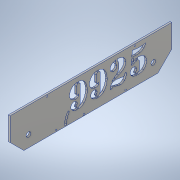
# Autodesk Inventor part: DriveTrain3.0
Saved by Autodesk Inventor 2021 (Build 250183000, 183)
## iProperties
Created: 2017-07-22
Part Number: DriveTrain3.0
Material: Aluminum 6061
Document SubType Name: Modeling
Designer: User
Density: 2.7 g/cm^3
Appearance: Aluminum - Flat
Mass: 590.045 g
Surface Area: 982.684 cm^2
Volume: 218.535 cm^3
Author: User
Autodesk Inventor part; units mm, degrees
ref_plane "YZ Plane" through (0, 0, 0) normal (1, 0, 0) x (0, 1, 0)
ref_plane "XZ Plane" through (0, 0, 0) normal (0, 1, 0) x (-1, 0, 0)
ref_plane "XY Plane" through (0, 0, 0) normal (0, 0, 1) x (1, 0, 0)
sketch "Sketch1" plane through (0, 0, 0) normal (1, 0, 0) x (0, 1, 0)
  line L0 (0, 0) -> (101.6, 0)
  line L1 (101.6, 0) -> (101.6, -444.5)
  line L2 (101.6, -444.5) -> (0, -444.5)
  line L3 (0, -444.5) -> (0, 0)
  circle A0 centre (31.75, -50.8) radius 6.3627
  circle A1 centre (31.75, -393.7) radius 6.3627
  circle A2 centre (86.2838, -165.5318) radius 1.5875
  circle A3 centre (70.2818, -165.5318) radius 1.5875
  circle A4 centre (15.3162, -278.9682) radius 1.5875
  circle A5 centre (31.3182, -278.9682) radius 1.5875
  dimension "d0" = 101.6
  dimension "d1" = 444.5
  dimension "d2" = 12.7254
  dimension "d3" = 31.75
  dimension "d4" = 50.8
  dimension "d5" = 50.8
  dimension "d22" = 165.5318
  dimension "d23" = 3.175
  dimension "d24" = 15.3162
  dimension "d25" = 3.175
  dimension "d26" = 16.002
  dimension "d27" = 165.5318
  dimension "d28" = 3.175
  dimension "d29" = 15.3162
  dimension "d30" = 165.5318
  dimension "d31" = 3.175
  dimension "d32" = 16.002
  dimension "d33" = 165.5318
  constraints: 8 end point, 6 centre point, 2 parallel, 1 horizontal, 1 perpendicular
  measures "d0" distance of L1.end L2.end
  measures "d1" distance of L0.end L1.end
  measures "d2" diameter of A0
  measures "d3" distance from line of L3 A0.centre
  measures "d4" distance from line of L0 A0.centre
  measures "d5" distance from line of L2 A1.centre
  measures "d22" distance from line of L0 A2.centre
  measures "d23" diameter of A2
  measures "d24" distance from line of L1 A2.centre
  measures "d25" diameter of A3
  measures "d26" distance of A2.centre A3.centre
  measures "d27" distance from line of L0 A3.centre
  measures "d28" diameter of A4
  measures "d29" distance from line of L3 A4.centre
  measures "d30" distance from line of L2 A4.centre
  measures "d31" diameter of A5
  measures "d32" distance of A5.centre A4.centre
  measures "d33" distance from line of L2 A5.centre
extrude "Extrusion1" add sketch "Sketch1" along normal blind 4.7625 contours L0 L1 L2 L3 | A2 | A3 | A4 | A5
chamfer "Chamfer1" distance 38.1 angle 45 1 edges at (2.3813, 0, 0)
chamfer "Chamfer2" distance 38.1 angle 45 1 edges at (2.3813, 0, -444.5)
sketch "Sketch8" plane through (4.7625, 0, 0) normal (1, 0, 0) x (0, 0, -1)
  line L0 (444.5, 38.1) -> (406.4, 0) projected
  line L1 (444.5, 38.1) -> (444.5, 101.6) projected
  line L2 (444.5, 101.6) -> (0, 101.6) projected
  line L3 (0, 101.6) -> (0, 38.1) projected
  line L4 (38.1, 0) -> (0, 38.1) projected
  line L5 (38.1, 0) -> (406.4, 0) projected
  circle A0 centre (393.7, 31.75) radius 6.3627 projected
  circle A1 centre (50.8, 31.75) radius 6.3627 projected
  point P0 (0, 0)
  point P1 (101.6, 97.155)
  point P2 (342.9, 97.155)
  point P3 (127, 4.445)
  point P4 (317.5, 4.445)
  dimension "d110" = 4.445
  dimension "d111" = 4.445
  dimension "d112" = 101.6
  dimension "d113" = 101.6
  dimension "d114" = 4.445
  dimension "d115" = 4.445
  dimension "d123" = 127
  dimension "d124" = 127
  measures "d110" distance from line of L2 point (342.9, 97.155)
  measures "d111" distance from line of L2 point (101.6, 97.155)
  measures "d112" distance from line of L3 point (101.6, 97.155)
  measures "d113" distance from line of L1 point (342.9, 97.155)
  measures "d114" distance from line of L5 point (317.5, 4.445)
  measures "d115" distance from line of L5 point (127, 4.445)
  measures "d123" distance from line of L1 point (317.5, 4.445)
  measures "d124" distance from line of L3 point (127, 4.445)
hole "Hole3" at (4.7625, 97.155, -101.6) at (4.7625, 97.155, -342.9) at (4.7625, 4.445, -127) at (4.7625, 4.445, -317.5) direction (-1, 0, 0) diameter 3.81 depth 25.4 tip angle 118
sketch "Sketch9" plane through (4.7625, 0, 0) normal (1, 0, 0) x (0, 0, -1)
  line L0 (444.5, 38.1) -> (444.5, 101.6) projected
  line L1 (38.1, 0) -> (406.4, 0) projected
  arc A0 (159.964, 30.48) -> (152.4159, 5.08) centre (203.2, 3.81) ccw construction
  arc A1 (157.8022, 31.8135) -> (149.8767, 5.1435) centre (203.2, 3.81) ccw
  arc A2 (162.1258, 29.1465) -> (154.9551, 5.0165) centre (203.2, 3.81) ccw
  arc A3 (162.1258, 29.1465) -> (157.8022, 31.8135) centre (159.964, 30.48) ccw
  arc A4 (149.8767, 5.1435) -> (154.9551, 5.0165) centre (152.4159, 5.08) ccw
  line L2 (0, 101.6) -> (0, 38.1) projected
  point P0 (0, 0)
  dimension "d126" = 3.81
  dimension "d134" = 50.8
  dimension "d135" = 5.08
  dimension "d238" = 203.2
  dimension "d239" = 5.08
  dimension "d240" = 25.4
  constraints: 10 point on circle, 5 centre point, 4 tangent, 1 coincident
  measures "d126" distance from line of point (203.2, 3.81) L1
  measures "d134" radius of A0
  measures "d135" diameter of A4
  measures "d238" distance from line of L2 point (203.2, 3.81)
  measures "d239" distance from line of A0.end L1
  measures "d240" vertical distance of A0.end A0.start
hole "Hole4" at (4.7625, 3.81, -203.2) direction (-1, 0, 0) diameter 5.08 end through all
extrude "Extrusion6" cut sketch "Sketch9" against normal through all
sketch "Sketch10" plane through (4.7625, 0, 0) normal (1, 0, 0) x (0, 0, -1)
  line L0 (161.1896, 89.2474) -> (414.9055, 89.2474) construction
  line L1 (414.9055, 89.2474) -> (414.9055, 0) construction
  line L2 (414.9055, 0) -> (161.1896, 0) construction
  line L3 (161.1896, 0) -> (161.1896, 89.2474) construction
  line L4 (188.4748, 24.204) -> (188.4748, 28.8893)
  spline S0 degree 2 poles (188.4748, 28.8893) (189.963, 29.3303) (191.5064, 30.3776) (192.0577, 31.3698) knots 0 0 0 1 2 2 2
  spline S1 degree 2 poles (192.0577, 31.3698) (193.2152, 33.299) (193.2152, 35.6141) knots 0 0 0 1 1 1
  line L5 (193.2152, 35.6141) -> (193.2152, 78.5538)
  spline S2 degree 2 poles (193.2152, 78.5538) (193.2152, 80.7036) (192.9396, 82.5226) (192.4435, 83.184) knots 0 0 0 1 2 2 2
  spline S3 degree 2 poles (192.4435, 83.184) (191.6718, 84.1211) (189.5772, 84.7274) knots 0 0 0 1 1 1
  line L6 (189.5772, 84.7274) -> (189.5772, 89.2474)
  spline S4 degree 2 poles (189.5772, 89.2474) (194.042, 88.8064) (201.8693, 84.4518) (204.901, 80.7587) knots 0 0 0 1 2 2 2
  spline S5 degree 2 poles (204.901, 80.7587) (208.3736, 76.6797) (212.1219, 63.8364) (212.1219, 56.3398) knots 0 0 0 1 2 2 2
  spline S6 degree 2 poles (212.1219, 56.3398) (212.1219, 40.3546) (202.9717, 31.0391) knots 0 0 0 1 1 1
  spline S7 degree 2 poles (202.9717, 31.0391) (199.7195, 27.7869) (192.1679, 24.204) (188.4748, 24.204) knots 0 0 0 1 2 2 2
  line L7 (189.5772, 59.3715) -> (189.5772, 54.0247)
  spline S8 degree 2 poles (189.5772, 54.0247) (184.506, 51.2687) (179.7656, 51.2687) knots 0 0 0 1 1 1
  spline S9 degree 2 poles (179.7656, 51.2687) (176.8441, 51.2687) (171.0564, 53.5286) (168.8515, 55.4579) knots 0 0 0 1 2 2 2
  spline S10 degree 2 poles (168.8515, 55.4579) (166.4261, 57.6628) (163.7252, 64.0569) (163.7252, 67.6949) knots 0 0 0 1 2 2 2
  spline S11 degree 2 poles (163.7252, 67.6949) (163.7252, 72.8763) (168.5208, 82.5777) (172.4895, 85.3338) knots 0 0 0 1 2 2 2
  spline S12 degree 2 poles (172.4895, 85.3338) (178.2221, 89.2474) (186.0494, 89.2474) knots 0 0 0 1 1 1
  line L8 (186.0494, 89.2474) -> (186.0494, 84.7274)
  spline S13 degree 2 poles (186.0494, 84.7274) (184.2304, 84.2313) (182.6319, 82.1918) (182.6319, 80.2075) knots 0 0 0 1 2 2 2
  line L9 (182.6319, 80.2075) -> (182.6319, 62.5134)
  spline S14 degree 2 poles (182.6319, 62.5134) (182.6319, 60.4188) (184.3958, 58.0486) (185.884, 58.1037) knots 0 0 0 1 2 2 2
  spline S15 degree 2 poles (185.884, 58.1037) (187.3172, 58.1588) (189.5772, 59.3715) knots 0 0 0 1 1 1
  line L10 (185.0021, 28.8893) -> (185.0021, 24.204)
  spline S16 degree 2 poles (185.0021, 24.204) (180.3719, 24.204) (175.6314, 26.4088) knots 0 0 0 1 1 1
  spline S17 degree 2 poles (175.6314, 26.4088) (171.6627, 28.3381) (167.1427, 34.4015) (167.1427, 37.9292) knots 0 0 0 1 2 2 2
  spline S18 degree 2 poles (167.1427, 37.9292) (167.1427, 41.7878) (172.3241, 47.0243) (176.2378, 47.0243) knots 0 0 0 1 2 2 2
  spline S19 degree 2 poles (176.2378, 47.0243) (179.7104, 47.0243) (184.5611, 42.5043) (184.5611, 39.3073) knots 0 0 0 1 2 2 2
  spline S20 degree 2 poles (184.5611, 39.3073) (184.5611, 37.1024) (183.5138, 35.559) knots 0 0 0 1 1 1
  line L11 (183.5138, 35.559) -> (182.0255, 33.4644)
  spline S21 degree 2 poles (182.0255, 33.4644) (181.4192, 32.5825) (181.4192, 31.8108) knots 0 0 0 1 1 1
  spline S22 degree 2 poles (181.4192, 31.8108) (181.4192, 30.4878) (182.8524, 29.4957) knots 0 0 0 1 1 1
  spline S23 degree 2 poles (182.8524, 29.4957) (183.5689, 28.9996) (185.0021, 28.8893) knots 0 0 0 1 1 1
  line L12 (243.2104, 24.204) -> (243.2104, 28.8893)
  spline S24 degree 2 poles (243.2104, 28.8893) (244.6987, 29.3303) (246.2421, 30.3776) (246.7933, 31.3698) knots 0 0 0 1 2 2 2
  spline S25 degree 2 poles (246.7933, 31.3698) (247.9509, 33.299) (247.9509, 35.6141) knots 0 0 0 1 1 1
  line L13 (247.9509, 35.6141) -> (247.9509, 78.5538)
  spline S26 degree 2 poles (247.9509, 78.5538) (247.9509, 80.7036) (247.6753, 82.5226) (247.1792, 83.184) knots 0 0 0 1 2 2 2
  spline S27 degree 2 poles (247.1792, 83.184) (246.4075, 84.1211) (244.3129, 84.7274) knots 0 0 0 1 1 1
  line L14 (244.3129, 84.7274) -> (244.3129, 89.2474)
  spline S28 degree 2 poles (244.3129, 89.2474) (248.7777, 88.8064) (256.605, 84.4518) (259.6366, 80.7587) knots 0 0 0 1 2 2 2
  spline S29 degree 2 poles (259.6366, 80.7587) (263.1093, 76.6797) (266.8576, 63.8364) (266.8576, 56.3398) knots 0 0 0 1 2 2 2
  spline S30 degree 2 poles (266.8576, 56.3398) (266.8576, 40.3546) (257.7074, 31.0391) knots 0 0 0 1 1 1
  spline S31 degree 2 poles (257.7074, 31.0391) (254.4552, 27.7869) (246.9036, 24.204) (243.2104, 24.204) knots 0 0 0 1 2 2 2
  line L15 (244.3129, 59.3715) -> (244.3129, 54.0247)
  spline S32 degree 2 poles (244.3129, 54.0247) (239.2417, 51.2687) (234.5012, 51.2687) knots 0 0 0 1 1 1
  spline S33 degree 2 poles (234.5012, 51.2687) (231.5798, 51.2687) (225.792, 53.5286) (223.5872, 55.4579) knots 0 0 0 1 2 2 2
  spline S34 degree 2 poles (223.5872, 55.4579) (221.1618, 57.6628) (218.4609, 64.0569) (218.4609, 67.6949) knots 0 0 0 1 2 2 2
  spline S35 degree 2 poles (218.4609, 67.6949) (218.4609, 72.8763) (223.2564, 82.5777) (227.2252, 85.3338) knots 0 0 0 1 2 2 2
  spline S36 degree 2 poles (227.2252, 85.3338) (232.9578, 89.2474) (240.7851, 89.2474) knots 0 0 0 1 1 1
  line L16 (240.7851, 89.2474) -> (240.7851, 84.7274)
  spline S37 degree 2 poles (240.7851, 84.7274) (238.9661, 84.2313) (237.3675, 82.1918) (237.3675, 80.2075) knots 0 0 0 1 2 2 2
  line L17 (237.3675, 80.2075) -> (237.3675, 62.5134)
  spline S38 degree 2 poles (237.3675, 62.5134) (237.3675, 60.4188) (239.1314, 58.0486) (240.6197, 58.1037) knots 0 0 0 1 2 2 2
  spline S39 degree 2 poles (240.6197, 58.1037) (242.0529, 58.1588) (244.3129, 59.3715) knots 0 0 0 1 1 1
  line L18 (239.7378, 28.8893) -> (239.7378, 24.204)
  spline S40 degree 2 poles (239.7378, 24.204) (235.1076, 24.204) (230.3671, 26.4088) knots 0 0 0 1 1 1
  spline S41 degree 2 poles (230.3671, 26.4088) (226.3984, 28.3381) (221.8784, 34.4015) (221.8784, 37.9292) knots 0 0 0 1 2 2 2
  spline S42 degree 2 poles (221.8784, 37.9292) (221.8784, 41.7878) (227.0598, 47.0243) (230.9735, 47.0243) knots 0 0 0 1 2 2 2
  spline S43 degree 2 poles (230.9735, 47.0243) (234.4461, 47.0243) (239.2968, 42.5043) (239.2968, 39.3073) knots 0 0 0 1 2 2 2
  spline S44 degree 2 poles (239.2968, 39.3073) (239.2968, 37.1024) (238.2495, 35.559) knots 0 0 0 1 1 1
  line L19 (238.2495, 35.559) -> (236.7612, 33.4644)
  spline S45 degree 2 poles (236.7612, 33.4644) (236.1549, 32.5825) (236.1549, 31.8108) knots 0 0 0 1 1 1
  spline S46 degree 2 poles (236.1549, 31.8108) (236.1549, 30.4878) (237.588, 29.4957) knots 0 0 0 1 1 1
  spline S47 degree 2 poles (237.588, 29.4957) (238.3046, 28.9996) (239.7378, 28.8893) knots 0 0 0 1 1 1
  line L20 (295.2452, 84.1762) -> (295.2452, 89.2474)
  line L21 (295.2452, 89.2474) -> (296.5129, 89.2474)
  spline S48 degree 2 poles (296.5129, 89.2474) (301.3636, 89.2474) (310.128, 86.0503) (313.0494, 83.184) knots 0 0 0 1 2 2 2
  spline S49 degree 2 poles (313.0494, 83.184) (318.0103, 78.3884) (318.0103, 71.1124) knots 0 0 0 1 1 1
  spline S50 degree 2 poles (318.0103, 71.1124) (318.0103, 64.8286) (310.6241, 55.1272) (303.789, 52.3711) knots 0 0 0 1 2 2 2
  line L22 (303.789, 52.3711) -> (297.7256, 49.9457)
  spline S51 degree 2 poles (297.7256, 49.9457) (295.0798, 48.8984) (290.2291, 46.2526) knots 0 0 0 1 1 1
  line L23 (290.2291, 46.2526) -> (288.8511, 45.4258)
  spline S52 degree 2 poles (288.8511, 45.4258) (286.9769, 45.4258) (283.5043, 44.4336) (280.2521, 43.0555) knots 0 0 0 1 2 2 2
  spline S53 degree 2 poles (280.2521, 43.0555) (281.9609, 45.3155) (285.3233, 48.5677) (288.7408, 51.2135) knots 0 0 0 1 2 2 2
  spline S54 degree 2 poles (288.7408, 51.2135) (293.0954, 54.5759) (296.1271, 57.6076) (297.2295, 59.6471) knots 0 0 0 1 2 2 2
  spline S55 degree 2 poles (297.2295, 59.6471) (298.2768, 61.6866) (299.269, 67.1988) (299.269, 71.4431) knots 0 0 0 1 2 2 2
  spline S56 degree 2 poles (299.269, 71.4431) (299.269, 78.8845) (297.9461, 81.4753) knots 0 0 0 1 1 1
  spline S57 degree 2 poles (297.9461, 81.4753) (297.45, 82.5226) (296.2925, 83.625) (295.2452, 84.1762) knots 0 0 0 1 2 2 2
  spline S58 degree 2 poles (317.5694, 45.6463) (318.6167, 45.7014) (319.9396, 43.9375) (319.9396, 42.5043) knots 0 0 0 1 2 2 2
  spline S59 degree 2 poles (319.9396, 42.5043) (319.9396, 39.2522) (316.5221, 31.3147) (314.1518, 28.8893) knots 0 0 0 1 2 2 2
  spline S60 degree 2 poles (314.1518, 28.8893) (312.1123, 26.7947) (306.1041, 24.204) (303.4031, 24.204) knots 0 0 0 1 2 2 2
  spline S61 degree 2 poles (303.4031, 24.204) (300.151, 24.204) (296.5129, 25.2513) knots 0 0 0 1 1 1
  line L24 (296.5129, 25.2513) -> (290.3945, 27.0703)
  spline S62 degree 2 poles (290.3945, 27.0703) (285.213, 28.5586) (283.6696, 28.5586) knots 0 0 0 1 1 1
  spline S63 degree 2 poles (283.6696, 28.5586) (281.6301, 28.5586) (279.3702, 26.6293) knots 0 0 0 1 1 1
  spline S64 degree 2 poles (279.3702, 26.6293) (277.937, 25.4167) (277.1653, 25.4167) knots 0 0 0 1 1 1
  spline S65 degree 2 poles (277.1653, 25.4167) (276.118, 25.4167) (274.9604, 26.7947) (274.9604, 28.1176) knots 0 0 0 1 2 2 2
  spline S66 degree 2 poles (274.9604, 28.1176) (274.9604, 30.5981) (277.2755, 35.8346) (279.2599, 37.7639) knots 0 0 0 1 2 2 2
  spline S67 degree 2 poles (279.2599, 37.7639) (283.5043, 41.898) (290.7803, 41.898) knots 0 0 0 1 1 1
  spline S68 degree 2 poles (290.7803, 41.898) (294.1978, 41.898) (299.9856, 40.8507) knots 0 0 0 1 1 1
  spline S69 degree 2 poles (299.9856, 40.8507) (308.3641, 39.2522) (310.8997, 39.2522) knots 0 0 0 1 1 1
  spline S70 degree 2 poles (310.8997, 39.2522) (313.1596, 39.2522) (314.207, 40.3546) knots 0 0 0 1 1 1
  spline S71 degree 2 poles (314.207, 40.3546) (314.5928, 40.7956) (315.0338, 41.8429) (315.3645, 43.276) knots 0 0 0 1 2 2 2
  spline S72 degree 2 poles (315.3645, 43.276) (315.8606, 45.536) (317.5694, 45.6463) knots 0 0 0 1 1 1
  line L25 (291.111, 89.1371) -> (291.111, 84.1762)
  spline S73 degree 2 poles (291.111, 84.1762) (289.7881, 83.9006) (288.1345, 82.9084) (288.1896, 82.3572) knots 0 0 0 1 2 2 2
  spline S74 degree 2 poles (288.1896, 82.3572) (288.2998, 81.7509) (289.4574, 80.9792) knots 0 0 0 1 1 1
  spline S75 degree 2 poles (289.4574, 80.9792) (291.552, 79.546) (293.4261, 76.1836) (293.4261, 73.8134) knots 0 0 0 1 2 2 2
  spline S76 degree 2 poles (293.4261, 73.8134) (293.4261, 70.2856) (288.0794, 65.1593) (284.4413, 65.1593) knots 0 0 0 1 2 2 2
  spline S77 degree 2 poles (284.4413, 65.1593) (280.4726, 65.1593) (275.1809, 70.6163) (275.1809, 74.6402) knots 0 0 0 1 2 2 2
  spline S78 degree 2 poles (275.1809, 74.6402) (275.1809, 78.4436) (279.8111, 85.0582) (283.7248, 86.9874) knots 0 0 0 1 2 2 2
  spline S79 degree 2 poles (283.7248, 86.9874) (286.2603, 88.2001) (291.111, 89.1371) knots 0 0 0 1 1 1
  line L26 (351.5242, 58.8754) -> (351.5242, 65.6003)
  spline S80 degree 2 poles (351.5242, 65.6003) (356.3198, 65.6003) (362.8241, 64.112) (365.8007, 62.3481) knots 0 0 0 1 2 2 2
  spline S81 degree 2 poles (365.8007, 62.3481) (375.1714, 56.8911) (375.1714, 45.3707) knots 0 0 0 1 1 1
  spline S82 degree 2 poles (375.1714, 45.3707) (375.1714, 39.8034) (370.8719, 30.9839) (366.9583, 28.2279) knots 0 0 0 1 2 2 2
  spline S83 degree 2 poles (366.9583, 28.2279) (364.1471, 26.4088) (356.7608, 24.204) (353.1228, 24.204) knots 0 0 0 1 2 2 2
  line L27 (353.1228, 24.204) -> (351.6345, 24.204)
  line L28 (351.6345, 24.204) -> (351.6345, 29.4405)
  spline S84 degree 2 poles (351.6345, 29.4405) (353.1228, 29.8815) (354.8315, 31.3698) (355.3827, 32.6376) knots 0 0 0 1 2 2 2
  spline S85 degree 2 poles (355.3827, 32.6376) (355.7686, 33.4093) (356.2647, 36.7166) (356.2647, 38.26) knots 0 0 0 1 2 2 2
  line L29 (356.2647, 38.26) -> (356.2647, 50.1662)
  spline S86 degree 2 poles (356.2647, 50.1662) (356.2647, 54.2452) (354.3354, 57.8281) (351.5242, 58.8754) knots 0 0 0 1 2 2 2
  line L30 (334.8224, 73.8685) -> (336.1453, 89.2474)
  spline S87 degree 2 poles (336.1453, 89.2474) (337.6887, 89.082) (337.9643, 89.0269) knots 0 0 0 1 1 1
  line L31 (337.9643, 89.0269) -> (347.335, 87.8142)
  spline S88 degree 2 poles (347.335, 87.8142) (352.3511, 87.0976) (359.2412, 87.0976) knots 0 0 0 1 1 1
  spline S89 degree 2 poles (359.2412, 87.0976) (363.9266, 87.0976) (369.6592, 88.0347) (372.8563, 89.2474) knots 0 0 0 1 2 2 2
  spline S90 degree 2 poles (372.8563, 89.2474) (371.8641, 86.0503) (369.549, 81.9713) (367.4544, 79.8767) knots 0 0 0 1 2 2 2
  spline S91 degree 2 poles (367.4544, 79.8767) (365.1944, 77.6167) (359.7925, 74.4748) (357.0915, 73.8685) knots 0 0 0 1 2 2 2
  spline S92 degree 2 poles (357.0915, 73.8685) (352.9574, 72.9314) (346.4531, 72.9314) knots 0 0 0 1 1 1
  spline S93 degree 2 poles (346.4531, 72.9314) (340.555, 72.9314) (334.8224, 73.8685) knots 0 0 0 1 1 1
  line L32 (347.6106, 29.4405) -> (347.6106, 24.3142)
  spline S94 degree 2 poles (347.6106, 24.3142) (342.7048, 24.645) (338.5156, 26.8498) knots 0 0 0 1 1 1
  spline S95 degree 2 poles (338.5156, 26.8498) (334.6019, 28.8893) (330.3576, 34.7873) (330.3576, 38.3151) knots 0 0 0 1 2 2 2
  spline S96 degree 2 poles (330.3576, 38.3151) (330.3576, 42.339) (335.539, 47.7409) (339.4526, 47.7409) knots 0 0 0 1 2 2 2
  spline S97 degree 2 poles (339.4526, 47.7409) (342.7599, 47.7409) (347.6657, 42.8902) (347.6657, 39.5829) knots 0 0 0 1 2 2 2
  spline S98 degree 2 poles (347.6657, 39.5829) (347.6657, 37.7088) (345.7916, 33.8503) (344.4687, 32.8581) knots 0 0 0 1 2 2 2
  spline S99 degree 2 poles (344.4687, 32.8581) (343.3662, 32.0312) (343.3662, 31.5352) knots 0 0 0 1 1 1
  spline S100 degree 2 poles (343.3662, 31.5352) (343.3662, 30.7634) (345.6262, 29.661) (347.6106, 29.4405) knots 0 0 0 1 2 2 2
  line L33 (334.4917, 70.2856) -> (338.7912, 69.8446)
  line L34 (338.7912, 69.8446) -> (337.9643, 60.1983)
  spline S101 degree 2 poles (337.9643, 60.1983) (340.7204, 62.4583) (345.0199, 64.7734) (347.6106, 65.4349) knots 0 0 0 1 2 2 2
  line L35 (347.6106, 65.4349) -> (347.6106, 58.8754)
  spline S102 degree 2 poles (347.6106, 58.8754) (342.6497, 57.7179) (339.2321, 55.6233) knots 0 0 0 1 1 1
  spline S103 degree 2 poles (339.2321, 55.6233) (337.0273, 54.2452) (335.98, 54.2452) knots 0 0 0 1 1 1
  spline S104 degree 2 poles (335.98, 54.2452) (334.7122, 54.2452) (333.279, 55.6233) (333.279, 56.7808) knots 0 0 0 1 2 2 2
  spline S105 degree 2 poles (333.279, 56.7808) (333.279, 57.332) (333.3341, 58.0486) knots 0 0 0 1 1 1
  line L36 (333.3341, 58.0486) -> (334.4917, 70.2856)
  point P0 (0, 0)
  constraints: 2 other
extrude "Extrusion7" cut sketch "Sketch10" against normal through all
equation "\"d110\" = d111"
equation "\"d112\" = d113"
equation "\"d114\" = d111"
equation "\"d115\" = d111"
equation "\"d124\" = d123"
body "Solid1"
